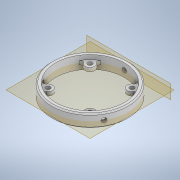
# Autodesk Inventor part: Electro_gps_2
Saved by Autodesk Inventor 2020 (Build 240168000, 168)
## iProperties
Created: 2020-09-03
Part Number: Electro_gps_2
Material: Generisch
Document SubType Name: Modeling
Designer: sp
Density: 1 g/cm^3
Appearance: Vorgabe
Author: sp
Autodesk Inventor part; units mm, degrees
ref_plane "YZ Plane" through (0, 0, 0) normal (1, 0, 0) x (0, 1, 0)
sketch "Skizze1" plane through (0, 0, 0) normal (0, 1, 0) x (-1, 0, 0)
  circle A0 centre (0, 0) radius 30
  circle A1 centre (0, 0) radius 27
  dimension "d0" = 60
  dimension "d1" = 54
  constraints: 2 centre point, 2 coincident
  measures "d0" diameter of A0
  measures "d1" diameter of A1
extrude "Extrusion1" add sketch "Skizze1" along normal mid plane 10
ref_plane "Arbeitsebene1" through (0, 0, 0) normal (0, 1, 0) x (-1, 0, 0)
chamfer "Fase1" distance 1 angle 45 2 edges at (30, 5, 0) (30, -5, 0)
sketch "Skizze2" plane through (0, 0, 0) normal (0, 1, 0) x (-1, 0, 0)
  line L0 (0, 42.2301) -> (0, -36.7007) construction
  line L1 (32.6355, 0) -> (-32.6355, 0) construction
  line L2 (16.5, 34.419) -> (16.5, -40.3324) construction
  line L3 (-16.5, 35.4304) -> (-16.5, -34.8157) construction
  line L4 (23.5881, 16.5) -> (-32.0387, 16.5) construction
  line L5 (23.5881, -16.5) -> (-39.8541, -16.5) construction
  circle A0 centre (16.5, -16.5) radius 1.75
  circle A1 centre (16.5, 16.5) radius 1.75
  circle A2 centre (-16.5, 16.5) radius 1.75
  circle A3 centre (-16.5, -16.5) radius 1.75
  circle A4 centre (-16.5, 16.5) radius 3.6749
  circle A5 centre (-16.5, -16.5) radius 3.7161
  circle A6 centre (16.5, -16.5) radius 3.7
  circle A7 centre (16.5, 16.5) radius 3.6747
  point P0 (0, 0)
  dimension "d8" = 33
  dimension "d9" = 33
  dimension "d10" = 3.5
  dimension "d11" = 3.5
  dimension "d12" = 3.5
  dimension "d13" = 3.5
  constraints: 12 end point, 9 point on line, 8 centre point, 4 coincident, 3 horizontal, 3 vertical, 1 midpoint, 2 other
  measures "d8" distance between parallel lines of L3 L2
  measures "d9" distance between parallel lines of L4 L5
  measures "d10" diameter of A0
  measures "d11" diameter of A1
  measures "d12" diameter of A2
  measures "d13" diameter of A3
extrude "Extrusion2" add sketch "Skizze2" along normal mid plane 3
fillet "Rundung1" radius 2 16 edges at (-18.7043, 0.75, -19.4718) (-19.4718, 0.75, -18.7043) (-18.7043, -0.75, -19.4718) (-19.4718, -0.75, -18.7043) (-19.289, 0.75, 18.8927) (-18.8927, 0.75, 19.289) (-19.289, -0.75, 18.8927) (-18.8927, -0.75, 19.289) (18.8904, 0.75, 19.2913) (19.2913, 0.75, 18.8904) (18.8904, -0.75, 19.2913) (19.2913, -0.75, 18.8904) (19.551, 0.75, -18.6215) (18.6215, 0.75, -19.551) (19.551, -0.75, -18.6215) (18.6215, -0.75, -19.551)
ref_plane "Arbeitsebene2" through (0, 0, -30.5) normal (0, 0, 1) x (1, 0, 0)
sketch "Skizze4" plane through (0, 0, -30.5) normal (0, 0, 1) x (1, 0, 0)
  circle A0 centre (0, 0) radius 1.75
  dimension "d27" = 3.5
  constraints: 1 centre point, 1 coincident
  measures "d27" diameter of A0
extrude "Extrusion4" cut sketch "Skizze4" along normal blind 5
pattern_circular "Runde Anordnung1" count 3 over 360 about axis through (0, -10, 0) along (0, 1, 0) of "Extrusion4"
